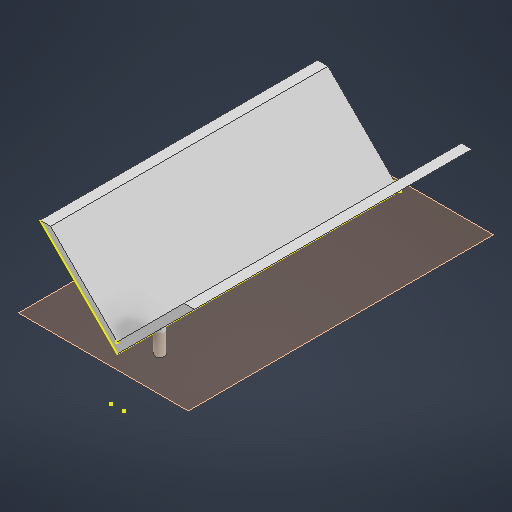
# Autodesk Inventor part: Part2
Saved by Autodesk Inventor 2026.2 (Build 302298010, 298A)
## iProperties
Created: 2026-04-05
Part Number: Part2
Material: Generic
Document SubType Name: Modeling
Designer: moham
Density: 1 g/cm^3
Appearance: Default
Author: moham
Autodesk Inventor part; units mm, degrees
ref_plane "YZ Plane" through (0, 0, 0) normal (1, 0, 0) x (0, 1, 0)
ref_plane "XZ Plane" through (0, 0, 0) normal (0, 1, 0) x (-1, 0, 0)
ref_plane "XY Plane" through (0, 0, 0) normal (0, 0, 1) x (1, 0, 0)
sketch "Sketch1" plane through (0, 0, 0) normal (0, 0, 1) x (1, 0, 0)
  point P0 (0, 0)
sketch "Sketch2" plane through (0, 0, 0) normal (0, 0, 1) x (1, 0, 0)
  line L0 (25, 25) -> (0, 0)
  line L1 (25, 25) -> (64.0581, 25) construction
  line L2 (-25, 25) -> (0, 0)
  line L3 (0, -5.6569) -> (34.6569, 29)
  line L4 (-34.6569, 29) -> (0, -5.6569)
  line L5 (25, 25) -> (29, 29)
  line L6 (-25, 25) -> (-29, 29)
  line L7 (29, 29) -> (36.0711, 36.0711)
  line L8 (-29, 29) -> (-36.0711, 36.0711)
  line L9 (34.6569, 29) -> (41.7279, 36.0711)
  line L10 (-34.6569, 29) -> (-41.7279, 36.0711)
  line L11 (-36.0711, 36.0711) -> (-41.7279, 36.0711)
  line L12 (36.0711, 36.0711) -> (41.7279, 36.0711)
  dimension "d2" = 135
  dimension "d3" = 0
  dimension "d4" = 4
  dimension "d13" = 59.0122
  dimension "d14" = 5.6569
  dimension "d15" = 11.0711
  dimension "d16" = 11.0711
  dimension "d17" = 4
  dimension "d18" = 25
  dimension "d19" = 23.6183
  dimension "d20" = 4
  dimension "d21" = 4
  dimension "d22" = 0
  dimension "d23" = 4
  dimension "d24" = 4
  dimension "d25" = 135
  constraints: 26 end point, 3 horizontal, 3 perpendicular, 2 parallel, 2 point on line
  measures "d2" angle of L0 L1
  measures "d3" distance of point (0, 0) L0.end
  measures "d4" distance between parallel lines of L0 L3
  measures "d13" distance of L3.start L10.end
  measures "d14" distance of L7.end L9.end
  measures "d15" distance between parallel lines of L1 L12
  measures "d16" distance between parallel lines of L1 L11
  measures "d17" distance between parallel lines of L4 L2
  measures "d18" distance from line of point (0, 0) L1
  measures "d19" distance from line of L1.end L9
  measures "d20" distance from line of L3.end L1
  measures "d21" distance from line of L5.end L1
  measures "d22" distance from line of L2.start L1
  measures "d23" distance from line of L6.end L1
  measures "d24" distance from line of L4.start L1
  measures "d25" angle of L6 L1
extrude "Extrusion1" add sketch "Sketch2" along normal blind 150
sketch "Sketch3" plane through (0, 0, 150) normal (0, 0, 1) x (1, 0, 0)
  line L0 (-41.7279, 36.0711) -> (0, -5.6569) projected
  point P0 (0, 0)
sketch "Sketch4" plane through (-36.0711, 36.0711, 0) normal (0.7071068, 0.7071068, 0) x (-0.7071068, 0.7071068, 0)
  point P0 (-51.0122, 0)
sketch "Sketch5" plane through (36.0711, 36.0711, 0) normal (0, 1, 0) x (1, 0, 0)
  line L0 (-72.1421, -150) -> (-77.799, -150) projected
  line L1 (-77.799, -150) -> (-77.799, -114)
  line L2 (-77.799, 0) -> (-77.799, -150) projected
  line L3 (-77.799, -114) -> (5.6569, -114)
  line L4 (5.6569, 0) -> (5.6569, -150) projected
  line L5 (5.6569, -107) -> (-77.799, -107)
  point P0 (-36.0711, 0)
  point P1 (5.6569, -107)
  dimension "d29" = 36
  dimension "d30" = 7
  constraints: 6 end point, 3 point on line, 1 perpendicular
  measures "d29" distance of L0.end L1.end
  measures "d30" distance between parallel lines of L3 L5
extrude "Extrusion2" cut sketch "Sketch5" against normal blind 41.728
sketch "Sketch6" plane through (0, 0, 150) normal (0, 0, 1) x (1, 0, 0)
  point P0 (0, 0)
sketch "Sketch7" plane through (36.0711, 36.0711, 107) normal (0, 0, 1) x (1, 0, 0)
  line L0 (5.6569, 0) -> (-36.0711, -41.7279) projected
  line L1 (-72.1421, 0) -> (-77.799, 0) projected
  line L2 (-36.0711, -41.7279) -> (-77.799, 0)
  line L3 (-77.799, 0) -> (-72.1421, 0)
  line L4 (-72.1421, 0) -> (-36.0711, -36.0711)
  line L5 (-36.0711, -36.0711) -> (0, 0)
  line L6 (0, 0) -> (5.6569, 0)
  line L7 (5.6569, 0) -> (-36.0711, -41.7279)
  constraints: 12 end point, 2 parallel, 2 point on line, 1 collinear, 1 perpendicular
extrude "Extrusion3" add sketch "Sketch7" along normal blind 10
sketch "Sketch9" plane through (0, -5.6569, 150) normal (0.7071068, -0.7071068, 0) x (-0.7071068, -0.7071068, 0)
  point P0 (-4, 150)
sketch "Sketch10" plane through (0, -5.6569, 150) normal (0.7071068, -0.7071068, 0) x (-0.7071068, -0.7071068, 0)
  line L0 (0, 150) -> (0, 0) projected
  point P0 (-4, 150)
  point P1 (0, 49.008)
  constraints: 1 point on line
sketch "Sketch16" plane through (0, 0, 150) normal (0, 0, 1) x (1, 0, 0)
  point P0 (-3.5, -30.6569)
  point P1 (3.5, -30.6569)
  point P2 (-3.5, -30.6569)
ref_plane "Work Plane3" through (0, -5.6569, 150) normal (0, 1, 0) x (1, 0, 0)
sketch "Sketch21" plane through (0, -5.6569, 150) normal (0, 1, 0) x (1, 0, 0)
  line L0 (0, 150) -> (0, 0) projected
  circle A0 centre (0, 23) radius 2.5
  line L1 (0, 23) -> (0, 0)
  dimension "d53" = 5
  dimension "d54" = 23
  constraints: 2 end point, 1 centre point, 1 collinear, 1 point on line
  measures "d53" diameter of A0
  measures "d54" distance of L0.end L1.start
extrude "Extrusion9" add sketch "Sketch21" along normal blind 5
sketch "Sketch22" plane through (0, -5.6569, 150) normal (0, -1, 0) x (1, 0, 0)
  circle A0 centre (0, -23) radius 2.5
  arc A1 (0, -20.5) -> (0, -25.5) centre (0, -23) ccw projected
  point P0 (0, -150)
  dimension "d57" = 5
  constraints: 1 centre point, 1 concentric
  measures "d57" diameter of A0
extrude "Extrusion10" add sketch "Sketch22" along normal blind 11.5
body "Solid1"
